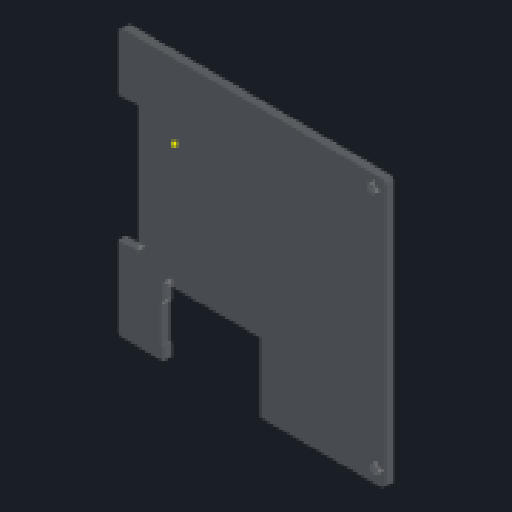
# Autodesk Inventor part: Lid_clear
Saved by Autodesk Inventor 2026.2 (Build 302298000, 298)
## iProperties
Created: 2026-04-26
Part Number: Lid_clear
Material: Generic
Document SubType Name: Modeling
Designer: Malthe Sennels
Density: 1 g/cm^3
Appearance: Polycarbonate - Clear
Author: Malthe Sennels
Autodesk Inventor part; units mm, degrees
ref_plane "YZ Plane" through (0, 0, 0) normal (1, 0, 0) x (0, 1, 0)
ref_plane "XZ Plane" through (0, 0, 0) normal (0, 1, 0) x (-1, 0, 0)
ref_plane "XY Plane" through (0, 0, 0) normal (0, 0, 1) x (1, 0, 0)
sketch "Sketch1" plane through (0, 0, 0) normal (0, 0, 1) x (1, 0, 0)
  line L0 (81.4908, -72.5941) -> (81.4908, 27.3941)
  line L1 (79.0849, 29.8) -> (81.4908, 27.3941)
  line L2 (-20.9033, 29.8) -> (79.0849, 29.8)
  line L3 (-23.3092, 27.3941) -> (-20.9033, 29.8)
  line L4 (-23.3092, -72.5941) -> (-23.3092, 27.3941)
  line L5 (-20.9033, -75) -> (-23.3092, -72.5941)
  line L6 (-4.3092, -75) -> (-20.9033, -75)
  line L7 (-4.3092, -73) -> (-4.3092, -75)
  line L8 (-4.3092, -73) -> (-20.0749, -73)
  line L9 (-21.3092, -71.7657) -> (-21.3092, 26.5657)
  line L10 (78.2565, 27.8) -> (-20.0749, 27.8)
  line L11 (79.4908, 26.5657) -> (78.2565, 27.8)
  line L12 (79.4908, -71.7657) -> (79.4908, 26.5657)
  line L13 (79.4908, -71.7657) -> (78.2565, -73)
  line L14 (78.2565, -73) -> (32.1708, -73)
  line L15 (32.1708, -75) -> (32.1708, -73)
  line L16 (79.0849, -75) -> (32.1708, -75)
  line L17 (79.0849, -75) -> (81.4908, -72.5941)
  line L18 (-4.3092, -75) -> (-23.3092, -75)
  line L19 (-23.3092, -75) -> (-23.3092, -73)
  line L20 (-23.3092, -73) -> (-4.3092, -73)
  line L21 (-4.3092, -73) -> (-4.3092, -75)
  line L22 (-21.3092, -59.0157) -> (-23.3092, -59.0157)
  line L23 (-23.3092, -59.0157) -> (-23.3092, -75)
  line L24 (-23.3092, -75) -> (-21.3092, -75)
  line L25 (-21.3092, -75) -> (-21.3092, -59.0157)
  line L26 (-20.9092, 18.65) -> (-20.9092, 26.4) construction
  line L27 (-20.9092, 26.4) -> (-19.9092, 27.4) construction
  line L28 (-19.9092, 27.4) -> (-12.1888, 27.4) construction
  line L29 (-21.3092, 18.65) -> (-21.3092, 26.5657)
  line L30 (-21.3092, 26.5657) -> (-20.0749, 27.8)
  line L31 (-20.0749, 27.8) -> (-12.1888, 27.8)
  line L32 (-22.7184, -70.3564) -> (-18.2476, -74.8272)
  line L33 (-22.7184, -70.3564) -> (-16.3958, -70.3564) construction
  line L34 (-4.3092, -75) -> (32.1708, -75)
  line L35 (32.1708, -75) -> (32.1708, -47)
  line L36 (32.1708, -47) -> (-4.3092, -47)
  line L37 (-4.3092, -47) -> (-4.3092, -75)
  circle A0 centre (-17.5342, -45.35) radius 1.75
  circle A1 centre (73.986, 22.4207) radius 1.75
  circle A2 centre (75.015, -68.5242) radius 1.75
  line L38 (-20.0749, -73) -> (-21.3092, -71.7657)
  line L39 (-21.3092, 26.5657) -> (-20.0749, 27.8)
  point P0 (0, 0)
  point P1 (-7.3249, -73)
  point P2 (-21.3092, -71.7657)
  point P3 (-20.0749, -73)
  point P4 (-17.9077, 27.8)
  point P5 (-21.3092, 18.65)
  point P6 (-21.3092, -74.5941)
extrude "Extrusion1" add sketch "Sketch1" against normal blind 3 contours L35 L36 L37 L8 L32 L9 L30 L10 L11 L12 L13 L14
sketch "Sketch2" plane through (0, 0, 0) normal (0, 0, 1) x (1, 0, 0)
  line L0 (-21.3092, -71.7657) -> (-21.3092, 26.5657) projected
  line L1 (-21.3092, 5.65) -> (-13.8092, 5.65)
  line L2 (-13.8092, 5.65) -> (-13.8092, -41.85)
  line L3 (-13.8092, -41.85) -> (-21.3092, -41.85)
  line L4 (-21.3092, -41.85) -> (-21.3092, 5.65)
  circle A0 centre (-17.5342, -45.35) radius 1.75 projected
  point P0 (0, 0)
  point P1 (-17.5592, 5.65)
  dimension "d6" = 7.5
  dimension "d7" = 3.5
  dimension "d8" = 47.5
  constraints: 8 end point, 2 parallel, 1 horizontal, 1 midpoint, 1 perpendicular, 1 point on line
  measures "d6" distance of L2.end L3.end
  measures "d7" distance from line of A0.centre L3
  measures "d8" distance from line of L3 point (-17.559, 5.65)
extrude "Extrusion2" cut sketch "Sketch2" against normal blind 3 contours L0 L1 L2 L3
sketch "Sketch3" plane through (0, 0, 0) normal (0, 0, 1) x (1, 0, 0)
  circle A0 centre (-17.5342, -45.35) radius 1.75 projected
  point P0 (0, 0)
extrude "Extrusion3" add sketch "Sketch3" against normal up to surface (3 mm away)
sketch "Sketch4" plane through (0, 0, 0) normal (0, 0, 1) x (1, 0, 0)
  line L0 (-3.3235, -61.1555) -> (-1.2915, -61.1555) projected
  line L1 (0.4425, -54.1555) -> (-5.0575, -54.1555)
  line L2 (-5.0575, -54.1555) -> (-5.0575, -68.1555)
  line L3 (-5.0575, -68.1555) -> (0.4425, -68.1555)
  line L4 (0.4425, -68.1555) -> (0.4425, -54.1555)
  line L5 (0.4425, -54.1555) -> (-5.0575, -68.1555) construction
  line L6 (-5.0575, -54.1555) -> (0.4425, -68.1555) construction
  point P0 (0, 0)
  point P1 (-2.3075, -61.1555)
  dimension "d13" = 5.5
  dimension "d14" = 14
  constraints: 12 end point, 3 midpoint, 2 parallel, 1 horizontal, 1 perpendicular
  measures "d13" distance of L3.end L2.end
  measures "d14" distance of L2.end L1.end
extrude "Extrusion4" cut sketch "Sketch4" against normal up to surface (3 mm away)
sketch "Sketch5" plane through (0, 0, 0) normal (0, 0, 1) x (1, 0, 0)
  point P0 (0, 0)
body "Solid1"
